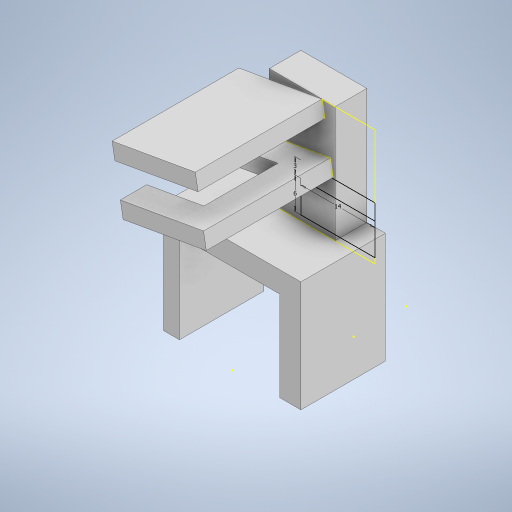
# Autodesk Inventor part: HolderMagasin
Saved by Autodesk Inventor 2023 (Build 270158000, 158)
## iProperties
Created: 2023-04-13
Part Number: HolderMagasin
Material: Generic
Document SubType Name: Modeling
Designer: Anders
Density: 1 g/cm^3
Appearance: Default
Author: Anders
## iProperties of the stored document HolderMagasin_3DPrint.ipt
Created: 2023-04-13
Part Number: HolderMagasin_3DPrint
Material: Generic
Document SubType Name: Modeling
Designer: Anders
Density: 1 g/cm^3
Appearance: Default
Author: Anders
Autodesk Inventor part; units mm, degrees
ref_plane "YZ Plane" through (0, 0, 0) normal (1, 0, 0) x (0, 1, 0)
ref_plane "XZ Plane" through (0, 0, 0) normal (0, 1, 0) x (-1, 0, 0)
ref_plane "XY Plane" through (0, 0, 0) normal (0, 0, 1) x (1, 0, 0)
sketch "Sketch1" plane through (0, 0, 0) normal (0, 1, 0) x (-1, 0, 0)
  line L0 (0, 0) -> (26, 0)
  line L1 (26, 0) -> (26, -33)
  line L2 (26, -33) -> (0, -33)
  line L3 (0, -33) -> (0, 0)
  dimension "d0" = 26
  dimension "d1" = 33
  constraints: 8 end point, 2 parallel, 1 horizontal, 1 perpendicular
  measures "d0" distance of L1.end L2.end
  measures "d1" distance of L0.end L1.end
extrude "Extrusion1" add sketch "Sketch1" along normal blind 4
sketch "Sketch2" plane through (0, 0, 0) normal (0, -1, 0) x (1, 0, 0)
  line L0 (-26, 0) -> (0, 0) projected
  line L1 (-26, -33) -> (-26, 0) projected
  line L2 (0, -33) -> (-26, -33) projected
  line L3 (0, 0) -> (0, -33) projected
  line L4 (-26, 0) -> (0, 0) projected
  line L5 (-26, -33) -> (-26, 0) projected
  line L6 (0, 0) -> (0, -33) projected
  line L7 (0, -33) -> (-26, -33) projected
  line L8 (0, 0) -> (-4, 0)
  line L9 (-4, 0) -> (-4, -33)
  line L10 (-4, -33) -> (0, -33)
  line L11 (0, -33) -> (0, 0)
  line L12 (-26, -33) -> (-26, 0) projected
  line L13 (-26, 0) -> (-23, 0)
  line L14 (-23, 0) -> (-23, -33)
  line L15 (-23, -33) -> (-26, -33)
  line L16 (-26, -33) -> (-26, 0)
  dimension "d4" = 4
  dimension "d5" = 3
  constraints: 16 end point, 4 parallel, 2 horizontal, 2 perpendicular, 2 point on line
  measures "d4" distance of L10.end L9.end
  measures "d5" distance of L14.end L15.end
extrude "Extrusion2" add sketch "Sketch2" along normal blind 17 contours L0 L14 L2 L1 | L0 L3 L2 L9
sketch "Sketch3" plane through (0, 4, 0) normal (0, 1, 0) x (1, 0, 0)
  line L0 (0, 33) -> (-26, 33) projected
  line L1 (-26, 33) -> (-26, 0) projected
  line L2 (-26, 0) -> (0, 0) projected
  line L3 (0, 0) -> (0, 33) projected
  line L4 (0, 0) -> (-6, 0)
  line L5 (-6, 0) -> (-6, 33)
  line L6 (-6, 33) -> (0, 33)
  line L7 (0, 33) -> (0, 0)
  line L8 (-6, 33) -> (-26, 33)
  line L9 (-26, 33) -> (-26, 27)
  line L10 (-26, 27) -> (-6, 27)
  line L11 (-6, 27) -> (-6, 33)
  dimension "d8" = 6
  dimension "d9" = 6
  constraints: 16 end point, 4 parallel, 2 horizontal, 2 perpendicular, 2 point on line
  measures "d8" distance of L5.end L6.end
  measures "d9" distance of L9.end L8.end
extrude "Extrusion3" add sketch "Sketch3" along normal blind 10 contours L5 L10 L1 L0
sketch "Sketch4" plane through (-26, 4, -27) normal (0, 0, 1) x (1, 0, 0)
  line L0 (20, 0) -> (0, 0) projected
  line L1 (20, 0) -> (20, 10) projected
  line L2 (0, 10) -> (20, 10) projected
  line L3 (0, 0) -> (0, 10) projected
  line L4 (20, 10) -> (6, 10)
  line L5 (6, 10) -> (6, 7)
  line L6 (6, 7) -> (20, 7)
  line L7 (20, 7) -> (20, 10)
  line L8 (20, 7) -> (6, 7)
  line L9 (6, 7) -> (6, 1)
  line L10 (6, 1) -> (20, 1)
  line L11 (20, 1) -> (20, 7)
  point P0 (26, -4)
  dimension "d12" = 14
  dimension "d13" = 3
  dimension "d14" = 6
  constraints: 16 end point, 4 parallel, 2 horizontal, 2 perpendicular, 1 point on line
  measures "d12" distance of L6.end L5.end
  measures "d13" distance of L5.end L4.end
  measures "d14" distance of L9.end L8.end
sketch "Sketch5" plane through (0, 14, 0) normal (0, 1, 0) x (1, 0, 0)
  line L0 (-6, 27) -> (-6, 33) projected
  line L1 (-6, 33) -> (-26, 33) projected
  line L2 (-26, 33) -> (-26, 27) projected
  line L3 (-26, 27) -> (-6, 27) projected
  line L4 (-26, 33) -> (-6, 33)
  line L5 (-6, 33) -> (-6, 27)
  line L6 (-6, 27) -> (-26, 27)
  line L7 (-26, 27) -> (-26, 33)
  point P0 (0, 0)
  constraints: 8 end point, 2 parallel, 1 horizontal, 1 perpendicular
extrude "Extrusion4" add sketch "Sketch5" along normal blind 12
sketch "Sketch6" plane through (-26, 4, -27) normal (0, 0, 1) x (1, 0, 0)
  line L0 (20, 0) -> (20, 22) projected
  line L1 (20, 22) -> (4.2431, 19.2216)
  line L2 (20, 22) -> (36, 22) construction
  line L3 (4.2431, 19.2216) -> (4.764, 16.2672)
  line L4 (4.764, 16.2672) -> (20.5209, 19.0456)
  line L5 (20.5209, 19.0456) -> (20, 22)
  line L6 (4.764, 16.2672) -> (5.8059, 10.3584)
  line L7 (5.8059, 10.3584) -> (6.3269, 7.4039)
  line L8 (6.3269, 7.4039) -> (22.0838, 10.1823)
  line L9 (22.0838, 10.1823) -> (21.5628, 13.1367)
  line L10 (21.5628, 13.1367) -> (5.8059, 10.3584)
  line L11 (20, 0) -> (0, 0) projected
  line L12 (20, 0) -> (20, 22) projected
  line L13 (0, 22) -> (20, 22) projected
  line L14 (0, 0) -> (0, 22) projected
  line L15 (0, -21) -> (0, 22) projected
  line L16 (20, 22) -> (10, 22)
  line L17 (20, 22) -> (0, 22) projected
  line L18 (10, 22) -> (-5.7569, 19.2216)
  line L19 (10, 22) -> (26, 22) construction
  line L20 (-5.7569, 19.2216) -> (-5.236, 16.2672)
  line L21 (-5.236, 16.2672) -> (10.5209, 19.0456)
  line L22 (10.5209, 19.0456) -> (10, 22)
  line L23 (-5.236, 16.2672) -> (-4.1941, 10.3584)
  line L24 (-5.236, 16.2672) -> (0.764, 16.2672) construction
  line L25 (-4.1941, 10.3584) -> (11.5628, 13.1367)
  line L26 (11.5628, 13.1367) -> (10.5209, 19.0456)
  line L27 (-4.1941, 10.3584) -> (-3.6731, 7.4039)
  line L28 (-4.1941, 10.3584) -> (-1.1941, 10.3584) construction
  line L29 (-3.6731, 7.4039) -> (12.0838, 10.1823)
  line L30 (12.0838, 10.1823) -> (11.5628, 13.1367)
  point P0 (26, -4)
  dimension "d17" = 16
  dimension "d18" = 170
  dimension "d19" = 3
  dimension "d20" = 6
  dimension "d21" = 3
  dimension "d22" = 16
  dimension "d27" = 16
  dimension "d28" = 170
  dimension "d29" = 16
  dimension "d30" = 6
  dimension "d31" = 80
  dimension "d32" = 3
  dimension "d33" = 80
  dimension "d34" = 16
  constraints: 48 end point, 10 perpendicular, 4 equal length, 4 horizontal, 3 parallel, 2 point on line, 1 midpoint
  measures "d17" distance of L0.end L1.end
  measures "d18" angle of L1 L2
  measures "d19" distance of L1.end L3.end
  measures "d20" distance of L3.end L6.end
  measures "d21" distance of L6.end L7.end
  measures "d22" distance of L7.end L8.end
  measures "d27" distance of L16.end L18.end
  measures "d28" angle of L18 L19
  measures "d29" distance of L20.end L21.end
  measures "d30" distance of L20.end L23.end
  measures "d31" angle of L23 L24
  measures "d32" distance of L23.end L27.end
  measures "d33" angle of L27 L28
  measures "d34" distance of L27.end L29.end
extrude "Extrusion5" add sketch "Sketch6" along normal blind 24 contours L29 L27 L25 L14 | L14 L25 L6 L7 L29 | L30 L29 L7 L10 | L10 L6 L25 L30 | L21 L20 L18 L14 | L14 L18 L22 L1 L3 L21 | L22 L21 L3 L1
sketch "Sketch7" plane through (-26, 4, 0) normal (0, 0, 1) x (1, 0, 0)
  line L0 (3, -4) -> (22, -4) projected
  line L1 (22, -4) -> (22, -21) projected
  line L2 (26, -21) -> (22, -21) projected
  line L3 (26, -21) -> (26, 0) projected
  line L4 (0, 0) -> (26, 0) projected
  line L5 (0, -21) -> (0, 0) projected
  line L6 (3, -21) -> (0, -21) projected
  line L7 (3, -4) -> (3, -21) projected
  line L8 (0, -21) -> (3, -21) projected
  line L9 (20, 0) -> (0, 0) projected
  line L10 (3, -21) -> (0, -21)
  line L11 (0, -21) -> (0, 0)
  line L12 (0, 0) -> (3, 0)
  line L13 (3, 0) -> (3, -21)
  line L14 (26, -4) -> (0, -4)
  line L15 (0, -4) -> (0, 0)
  line L16 (0, 0) -> (26, 0)
  line L17 (26, 0) -> (26, -4)
  line L18 (22, -4) -> (22, -21) projected
  line L19 (26, -4) -> (22, -4)
  line L20 (22, -4) -> (22, -21)
  line L21 (22, -21) -> (26, -21)
  line L22 (26, -21) -> (26, -4)
  constraints: 24 end point, 6 parallel, 3 horizontal, 3 perpendicular
extrude "Extrusion6" cut sketch "Sketch7" against normal blind 17
sketch "Sketch8" plane through (-26, 4, -27) normal (0, 0, 1) x (1, 0, 0)
  line L0 (11.5628, 13.1367) -> (-4.1941, 10.3584) projected
  line L1 (-4.1941, 10.3584) -> (-3.6731, 7.4039) projected
  line L2 (-3.6731, 7.4039) -> (12.0838, 10.1823) projected
  line L3 (12.0838, 10.1823) -> (11.5628, 13.1367) projected
  line L4 (12.0838, 10.1823) -> (0, 8.0516) projected
  line L5 (0, 0) -> (0, 8.0516) projected
  line L6 (20, 0) -> (0, 0) projected
  line L7 (20, 0) -> (20, 22) projected
  line L8 (10, 22) -> (20, 22) projected
  line L9 (10, 22) -> (10.5209, 19.0456) projected
  line L10 (10.5209, 19.0456) -> (0, 17.1905) projected
  line L11 (0, 11.0979) -> (0, 17.1905) projected
  line L12 (0, 11.0979) -> (11.5628, 13.1367) projected
  line L13 (11.5628, 13.1367) -> (12.0838, 10.1823) projected
  point P0 (26, -4)
sketch "Sketch9" plane through (-26, -17, -33) normal (-1, 0, 0) x (0, 0, 1)
  line L0 (16, 0) -> (16, 21) projected
  line L1 (6, 21) -> (16, 21) projected
  line L2 (6, 21) -> (6, 29.0516) projected
  line L3 (6, 29.0516) -> (6, 32.0979) projected
  line L4 (6, 32.0979) -> (6, 38.1905) projected
  line L5 (6, 38.1905) -> (6, 41.2367) projected
  line L6 (6, 41.2367) -> (6, 43) projected
  line L7 (0, 43) -> (6, 43) projected
  line L8 (0, 0) -> (0, 43) projected
  line L9 (16, 0) -> (0, 0) projected
  line L10 (0, 17) -> (0, 0) projected
  line L11 (16, 21) -> (0, 21)
  line L12 (0, 21) -> (0, 0)
  line L13 (0, 0) -> (16, 0)
  line L14 (16, 0) -> (16, 21)
  point P0 (33, 17)
  constraints: 8 end point, 2 parallel, 1 horizontal, 1 perpendicular
sketch "Sketch10" plane through (-4, -17, -33) normal (-1, 0, 0) x (0, 0, 1)
  line L0 (16, 0) -> (16, 17) projected
  line L1 (0, 17) -> (16, 17) projected
  line L2 (0, 17) -> (0, 0) projected
  line L3 (16, 0) -> (0, 0) projected
  line L4 (16, 17) -> (0, 17)
  line L5 (0, 17) -> (0, 0)
  line L6 (0, 0) -> (16, 0)
  line L7 (16, 0) -> (16, 17)
  point P0 (33, 17)
  constraints: 8 end point, 2 parallel, 1 horizontal, 1 perpendicular
sketch "Sketch11" plane through (-23, -17, -33) normal (1, 0, 0) x (0, 0, -1)
  line L0 (-16, 17) -> (-16, 0) projected
  line L1 (0, 0) -> (-16, 0) projected
  line L2 (0, 17) -> (0, 0) projected
  line L3 (-16, 17) -> (0, 17) projected
  line L4 (-16, 17) -> (0, 17)
  line L5 (0, 17) -> (0, 0)
  line L6 (0, 0) -> (-16, 0)
  line L7 (-16, 0) -> (-16, 17)
  point P0 (-33, 17)
  constraints: 8 end point, 2 parallel, 1 horizontal, 1 perpendicular
sketch "Sketch12" plane through (0, -17, -33) normal (1, 0, 0) x (0, 0, -1)
  line L0 (-16, 21) -> (-16, 0) projected
  line L1 (0, 0) -> (-16, 0) projected
  line L2 (0, 21) -> (0, 0) projected
  line L3 (-16, 21) -> (0, 21) projected
  line L4 (0, 17) -> (-16, 17) projected
  line L5 (-16, 21) -> (0, 21)
  line L6 (0, 21) -> (0, 0)
  line L7 (0, 0) -> (-16, 0)
  line L8 (-16, 0) -> (-16, 21)
  point P0 (-33, 17)
  constraints: 8 end point, 2 parallel, 1 horizontal, 1 perpendicular
extrude "Extrusion7" add sketch "Sketch10" along normal blind 10
extrude "Extrusion8" cut sketch "Sketch12" against normal blind 10
extrude "Extrusion9" add sketch "Sketch9" along normal blind 10 contours L9 L8 L11 L1 L0
extrude "Extrusion10" cut sketch "Sketch11" against normal blind 10
sketch "Sketch13" plane through (-26, 4, -17) normal (0, 0, 1) x (1, 0, 0)
  point P0 (26, -4)
sketch "Sketch15" plane through (-13.9162, 14.1823, -27) normal (0.1736482, -0.9848078, 0) x (0.9848078, 0.1736482, 0)
  line L0 (-16, 0) -> (-12.2702, 0) projected
  line L1 (0, 0) -> (-12.2702, 0) projected
  line L2 (0, 0) -> (0, 24) projected
  line L3 (-16, 24) -> (0, 24) projected
  line L4 (-16, 0) -> (-16, 24) projected
  line L5 (-16, 0) -> (-16, 5)
  line L6 (-16, 24) -> (-16, 19)
  line L7 (-16, 24) -> (-11, 24) construction
  line L8 (-16, 19) -> (-5, 19)
  line L9 (-5, 19) -> (-5, 5)
  line L10 (-5, 5) -> (-16, 5)
  line L11 (-16, 5) -> (-16, 19)
  point P0 (11.2421, 27)
  dimension "d43" = 5
  dimension "d44" = 5
  dimension "d45" = 90
  dimension "d46" = 11
  constraints: 14 end point, 2 horizontal, 2 parallel, 2 perpendicular, 1 collinear, 1 point on line
  measures "d43" distance of L0.start L5.end
  measures "d44" distance of L3.start L6.end
  measures "d45" angle of L6 L7
  measures "d46" distance of L9.end L10.end
extrude "Extrusion11" cut sketch "Sketch15" against normal blind 4 contours L4 L8 L9 L10
sketch "Sketch16" plane through (-6, 26, -27) normal (1, 0, 0) x (0, 0, -1)
  point P0 (-27, -26)
sketch "Sketch17" plane through (-6, 26, -27) normal (1, 0, 0) x (0, 0, -1)
  line L0 (6, -22) -> (0, -22) projected
  line L1 (6, -22) -> (6, 0) projected
  line L2 (0, 0) -> (6, 0) projected
  line L3 (0, -22) -> (0, 0) projected
  line L4 (0, 0) -> (6, 0)
  line L5 (6, 0) -> (6, -22)
  line L6 (6, -22) -> (0, -22)
  line L7 (0, -22) -> (0, 0)
  point P0 (-27, -26)
  constraints: 8 end point, 2 parallel, 1 horizontal, 1 perpendicular
extrude "Extrusion12" cut sketch "Sketch17" against normal blind 7.5
body "Solid1"
